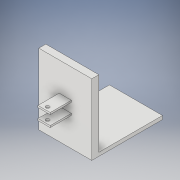
# Autodesk Inventor part: LucasCharles Part3
Saved by Autodesk Inventor 2018 (Build 220112000, 112)
## iProperties
Created: 2018-05-15
Part Number: LucasCharles Part3
Material: ABS Plastic
Document SubType Name: Modeling
Designer: 21lsilva
Density: 1.06 g/cm^3
Appearance: Smooth - White
Author: 21lsilva
Autodesk Inventor part; units mm, degrees
ref_plane "YZ Plane" through (0, 0, 0) normal (1, 0, 0) x (0, 1, 0)
ref_plane "XZ Plane" through (0, 0, 0) normal (0, 1, 0) x (-1, 0, 0)
ref_plane "XY Plane" through (0, 0, 0) normal (0, 0, 1) x (1, 0, 0)
sketch "Sketch1" plane through (0, 0, 0) normal (0, 0, 1) x (1, 0, 0)
  line L0 (0, 0) -> (190.5, 0)
  line L1 (190.5, 0) -> (190.5, 254)
  line L2 (190.5, 254) -> (0, 254)
  line L3 (0, 254) -> (0, 0)
  dimension "d0" = 190.5
  dimension "d1" = 254
  constraints: 8 end point, 2 parallel, 1 horizontal, 1 perpendicular
  measures "d0" distance of L2.end L1.end
  measures "d1" distance of L1.end L0.end
extrude "Extrusion1" add sketch "Sketch1" against normal blind 25.4
sketch "Sketch2" plane through (0, 0, 0) normal (0, 0, 1) x (1, 0, 0)
  line L0 (0, 0) -> (0, 254) projected
  line L1 (0, 127) -> (190.5, 127)
  line L2 (190.5, 254) -> (190.5, 0) projected
  line L3 (54.1274, 112.395) -> (54.1274, 106.045)
  line L4 (95.25, 144.145) -> (117.3226, 144.145)
  line L5 (117.3226, 144.145) -> (73.1774, 144.145)
  line L6 (95.25, 109.855) -> (117.3226, 109.855)
  line L7 (117.3226, 109.855) -> (73.1774, 109.855)
  line L8 (73.1774, 144.145) -> (117.3226, 144.145)
  line L9 (117.3226, 144.145) -> (117.3226, 150.495)
  line L10 (117.3226, 150.495) -> (73.1774, 150.495)
  line L11 (73.1774, 150.495) -> (73.1774, 144.145)
  line L12 (73.1774, 109.855) -> (117.3226, 109.855)
  line L13 (117.3226, 109.855) -> (117.3226, 103.505)
  line L14 (117.3226, 103.505) -> (73.1774, 103.505)
  line L15 (73.1774, 103.505) -> (73.1774, 109.855)
  point P0 (54.1274, 141.605)
  dimension "d16" = 22.0726
  dimension "d17" = 44.1452
  dimension "d18" = 6.35
  dimension "d19" = 6.35
  constraints: 28 end point, 4 parallel, 4 symmetric about line, 3 horizontal, 2 midpoint, 2 perpendicular, 2 point on line
  measures "d16" distance of L4.start L4.end
  measures "d17" distance of L4.end L5.end
  measures "d18" distance of L9.end L8.end
  measures "d19" distance of L12.end L13.end
extrude "Extrusion2" add sketch "Sketch2" along normal blind 76.2
sketch "Sketch3" plane through (54.1274, 112.395, 0) normal (0, 1, 0) x (1, 0, 0)
  circle A0 centre (22.0726, -63.5) radius 6.35
  point P0 (-54.1274, 0)
  dimension "d10" = 12.7
  constraints: 1 centre point, 1 coincident
  measures "d10" diameter of A0
extrude "Extrusion3" [suppressed]
sketch "Sketch4" plane through (0, 0, -25.4) normal (0, 0, -1) x (-1, 0, 0)
  line L0 (-190.5, 0) -> (-190.5, 254) projected
  line L1 (0, 0) -> (-190.5, 0)
  line L2 (-190.5, 0) -> (-190.5, 12.7)
  line L3 (-190.5, 12.7) -> (0, 12.7)
  line L4 (0, 12.7) -> (0, 0)
  dimension "d13" = 12.7
  constraints: 8 end point, 2 parallel, 1 horizontal, 1 perpendicular, 1 point on line
  measures "d13" distance of L1.end L2.end
extrude "Extrusion4" add sketch "Sketch4" along normal blind 228.6
sketch "Sketch5" plane through (73.1774, 150.495, 0) normal (0, 1, 0) x (1, 0, 0)
  circle A0 centre (22.0726, -63.5) radius 6.35
  point P0 (-73.1774, 0)
  dimension "d20" = 12.7
  constraints: 1 centre point, 1 coincident
  measures "d20" diameter of A0
extrude "Extrusion5" cut sketch "Sketch5" against normal blind 101.6
body "Solid1"
